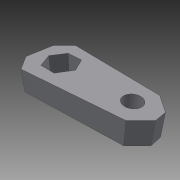
# Autodesk Inventor part: y_carriage_nut_holder_b
Saved by Autodesk Inventor 2014 (Build 180170000, 170)
## iProperties
Created: 2013-12-05
Part Number: y_carriage_nut_holder_b
Material: Generic
Document SubType Name: Modeling
Designer: buben
Density: 1 g/cm^3
Appearance: Anodized - Dark Gray
Author: buben
Subject: Laser Cutted
Autodesk Inventor part; units mm, degrees
ref_plane "YZ Plane" through (0, 0, 0) normal (1, 0, 0) x (0, 1, 0)
ref_plane "XZ Plane" through (0, 0, 0) normal (0, 1, 0) x (-1, 0, 0)
ref_plane "XY Plane" through (0, 0, 0) normal (0, 0, 1) x (1, 0, 0)
sketch "Sketch1" plane through (0, 0, 0) normal (0, 0, 1) x (1, 0, 0)
  line L0 (-4, -8) -> (22.5, -5)
  line L1 (26, -1.5) -> (26, 1.5)
  line L2 (22.5, 5) -> (-4, 8)
  line L3 (-8, 4) -> (-8, -4)
  line L4 (-4, 8) -> (-8, 4)
  line L5 (-8, -4) -> (-4, -8)
  line L6 (22.5, -5) -> (26, -1.5)
  line L7 (26, 1.5) -> (22.5, 5)
  circle A0 centre (0, 0) radius 2.75
  circle A1 centre (20, 0) radius 2.25
  circle A2 centre (0, 0) radius 5 construction
  circle A3 centre (20, 0) radius 4.5 construction
  point P0 (-8, 0)
  point P1 (26, 0)
  dimension "d9" = 8
  dimension "d10" = 20
  dimension "d11" = 4.5
  dimension "d12" = 5.5
  dimension "d13" = 6
  dimension "d16" = 10
  dimension "d17" = 9
  dimension "d18" = 8
  dimension "d19" = 4
  dimension "d20" = 4
  dimension "d21" = 4
  dimension "d22" = 10
  dimension "d23" = 3
  constraints: 16 end point, 4 centre point, 3 horizontal alignment, 3 parallel, 2 coincident, 2 midpoint, 2 perpendicular, 1 vertical alignment, 1 other
  measures "d9" distance from line of L3 A0.centre
  measures "d10" distance of A1.centre A0.centre
  measures "d11" diameter of A1
  measures "d12" diameter of A0
  measures "d13" distance from line of L1 A1.centre
  measures "d16" diameter of A2
  measures "d17" diameter of A3
  measures "d18" distance of L3.start L3.end
  measures "d19" horizontal distance of L0.start L3.end
  measures "d20" horizontal distance of L2.end L3.start
  measures "d21" horizontal distance of L2.end L3.start
  measures "d22" distance of L0.end L2.start
  measures "d23" distance of L1.start L1.end
extrude "Extrusion1" add sketch "Sketch1" along normal blind 6
sketch "Sketch2" plane through (0, 0, 6) normal (0, 0, 1) x (1, 0, 0)
  circle A0 centre (0, 0) radius 2.75 projected
  line L0 (-8, 4) -> (-8, -4) projected
  line L1 (4.6188, 0) -> (2.3094, -4)
  line L2 (2.3094, -4) -> (-2.3094, -4)
  line L3 (-2.3094, -4) -> (-4.6188, 0)
  line L4 (-4.6188, 0) -> (-2.3094, 4)
  line L5 (-2.3094, 4) -> (2.3094, 4)
  line L6 (2.3094, 4) -> (4.6188, 0)
  dimension "d24" = 8
  constraints: 12 end point, 1 coincident, 1 perpendicular, 13 other
  measures "d24" distance between parallel lines of L2 L5
extrude "Extrusion2" cut sketch "Sketch2" against normal through all
body "Solid1"
